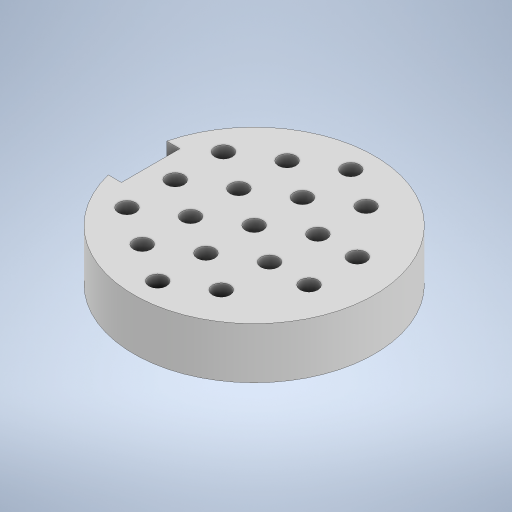
# Autodesk Inventor part: male
Saved by Autodesk Inventor 2023 (Build 270158000, 158)
## iProperties
Created: 2022-10-21
Part Number: male
Material: Generic
Document SubType Name: Modeling
Designer: rayle
Density: 1 g/cm^3
Appearance: Default
Author: rayle
Autodesk Inventor part; units mm, degrees
ref_plane "YZ Plane" through (0, 0, 0) normal (1, 0, 0) x (0, 1, 0)
ref_plane "XZ Plane" through (0, 0, 0) normal (0, 1, 0) x (-1, 0, 0)
ref_plane "XY Plane" through (0, 0, 0) normal (0, 0, 1) x (1, 0, 0)
sketch "Sketch1" plane through (0, 0, 0) normal (0, 1, 0) x (-1, 0, 0)
  point P0 (0, 0)
sketch "Sketch3" plane through (0, 0, 0) normal (0, 1, 0) x (-1, 0, 0)
  circle A0 centre (0, 0) radius 8.2273
  line L0 (0, 0) -> (7.55, 0)
  line L1 (7.55, -2) -> (7.9805, -2)
  line L2 (7.55, 1.9983) -> (7.9813, 1.9967)
  circle A1 centre (-2.7, -1.65) radius 0.6
  line L3 (-2.7, -4.35) -> (-2.7, -4.95)
  circle A2 centre (-2.7, -4.95) radius 0.6
  line L4 (0, -0.6) -> (0, -1.65)
  line L5 (0, -0.6) -> (0, -1.65)
  circle A3 centre (0, 0) radius 0.6
  circle A4 centre (-5.4, -1.65) radius 0.6
  line L6 (-2.7, 1.65) -> (-5.4, 1.65)
  circle A5 centre (-5.4, 1.65) radius 0.6
  line L7 (0, 0.6) -> (0, 3.3)
  circle A6 centre (0, 3.3) radius 0.6
  circle A7 centre (-2.7, 1.65) radius 0.6
  line L8 (-2.7, 1.65) -> (-2.7, 4.95)
  circle A8 centre (-2.7, 4.95) radius 0.6
  line L9 (0, 3.9) -> (0, 6.6)
  circle A9 centre (0, 6.6) radius 0.6
  circle A10 centre (5.4, 0) radius 0.6
  line L10 (2.7, 1.05) -> (2.7, 1.65)
  circle A11 centre (2.7, 1.65) radius 0.6
  line L11 (5.4, 0) -> (5.4, 3.3)
  circle A12 centre (5.4, 3.3) radius 0.6
  line L12 (2.7, 2.25) -> (2.7, 4.95)
  circle A13 centre (2.7, 4.95) radius 0.6
  line L13 (0, -2.7) -> (0, -3.3)
  circle A14 centre (0, -3.3) radius 0.6
  line L14 (0, -3.9) -> (0, -6)
  line L15 (0, -6) -> (0, -6.6)
  circle A15 centre (0, -6.6) radius 0.6
  line L16 (2.7, 0) -> (5.4, 0)
  circle A16 centre (2.7, -1.65) radius 0.6
  line L17 (5.4, 0) -> (5.4, -3.3)
  circle A17 centre (5.4, -3.3) radius 0.6
  line L18 (2.7, -3.75) -> (2.7, -4.95)
  circle A18 centre (2.7, -4.95) radius 0.6
  line L19 (2.7, -1.65) -> (2.7, -3.75)
  line L20 (8.2273, 0.0003) -> (7.0773, 0)
  line L21 (7.0773, 0) -> (7.0773, 2)
  line L22 (7.0773, 2) -> (7.55, 1.9983)
  line L23 (7.0773, 0) -> (7.0773, -2)
  line L24 (7.0773, -2) -> (7.55, -2)
  dimension "d10" = 1.2
  dimension "d15" = 1.2
  dimension "d26" = 1.2
  dimension "d3" = 2
  dimension "d7" = 1.2
  dimension "d8" = 2.1
  dimension "d9" = 0.6
  dimension "d11" = 2.1
  dimension "d12" = 0.6
  dimension "d13" = 1.2
  dimension "d14" = 2.7
  dimension "d16" = 2.7
  dimension "d17" = 1.2
  dimension "d18" = 1.05
  dimension "d20" = 1.2
  dimension "d21" = 2.1
  dimension "d22" = 1.2
  dimension "d23" = 1.2
  dimension "d25" = 0.6
  dimension "d27" = 2.7
  dimension "d28" = 1.2
  dimension "d29" = 2.7
  dimension "d30" = 1.2
  dimension "d31" = 1.2
  dimension "d32" = 1.2
  dimension "d34" = 1.2
  dimension "d35" = 2.7
  dimension "d36" = 0.6
  dimension "d37" = 1.2
  dimension "d38" = 1.2
  dimension "d39" = 1.2
  dimension "d42" = 2.7
  dimension "d46" = 1.15
  dimension "d47" = 2
  dimension "d48" = 2
  constraints: 50 end point, 16 centre point, 14 coincident, 10 vertical, 5 point on circle, 3 vertical alignment, 2 horizontal, 2 perpendicular, 1 collinear, 1 point on line, 6 other
  measures "d3" distance of L0.end L1.start
  measures "d7" diameter of A3
  measures "d8" distance of L4.start L13.start
  measures "d9" distance of L13.start L13.end
  measures "d11" distance of L14.start L14.end
  measures "d12" distance of L14.end L15.end
  measures "d13" diameter of A15
  measures "d14" distance of L7.start L7.end
  measures "d16" distance of L9.start L9.end
  measures "d17" diameter of A9
  measures "d18" distance of L4.start L4.end
  measures "d20" diameter of A16
  measures "d21" distance of L19.start L19.end
  measures "d22" distance of L19.end L18.end
  measures "d23" diameter of A18
  measures "d25" distance of L10.start L10.end
  measures "d27" distance of L12.start L12.end
  measures "d28" diameter of A13
  measures "d29" distance of L16.start L16.end
  measures "d30" diameter of A10
  measures "d31" diameter of A17
  measures "d32" diameter of A12
  measures "d34" diameter of A1
  measures "d35" distance of A1.centre L3.start
  measures "d36" distance of L3.start L3.end
  measures "d37" diameter of A2
  measures "d38" diameter of A7
  measures "d39" diameter of A8
  measures "d42" distance of L8.start L6.end
  measures "d46" distance of L20.start L20.end
  measures "d47" distance of L20.end L21.end
  measures "d48" distance of L20.end L23.end
extrude "Extrusion1" add sketch "Sketch3" along normal blind 3.5 contours L2 L22 L21 L23 L24 L1 A0
body "Solid1"
